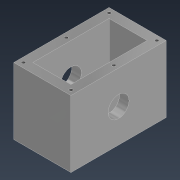
# Autodesk Inventor part: P016-Carter_corps
Saved by Autodesk Inventor 2021.3 (Build 253353000, 353)
## iProperties
Created: 2022-04-01
Part Number: P016-Carter_corps
Material: Aluminium
Document SubType Name: Modeling
Designer: remi
Density: 2.7 g/cm^3
Appearance: Aluminum - Dark
Author: remi
Autodesk Inventor part; units mm, degrees
ref_plane "YZ Plane" through (0, 0, 0) normal (1, 0, 0) x (0, 1, 0)
ref_plane "XZ Plane" through (0, 0, 0) normal (0, 1, 0) x (-1, 0, 0)
ref_plane "XY Plane" through (0, 0, 0) normal (0, 0, 1) x (1, 0, 0)
sketch "Sketch2" plane through (0, 0, 0) normal (0, 0, 1) x (1, 0, 0)
  line L0 (-30, -50) -> (30, -50)
  line L1 (30, -50) -> (30, 50)
  line L2 (30, 50) -> (-30, 50)
  line L3 (-30, 50) -> (-30, -50)
  line L4 (-30, -50) -> (30, 50) construction
  line L5 (30, -50) -> (-30, 50) construction
  line L6 (20, -40) -> (-20, -40)
  line L7 (-20, -40) -> (-20, 40)
  line L8 (-20, 40) -> (20, 40)
  line L9 (20, 40) -> (20, -40)
  line L10 (20, -40) -> (-20, 40) construction
  line L11 (-20, -40) -> (20, 40) construction
  point P0 (0, 0)
  dimension "d0" = 60
  dimension "d1" = 10
  dimension "d2" = 10
  dimension "d3" = 80
  constraints: 24 end point, 4 midpoint, 4 parallel, 2 horizontal, 2 perpendicular
  measures "d0" distance of L1.end L2.end
  measures "d1" distance between parallel lines of L3 L7
  measures "d2" distance between parallel lines of L2 L8
  measures "d3" distance of L6.end L7.end
extrude "Extrusion1" add sketch "Sketch2" along normal blind 60
sketch "Sketch3" plane through (0, 0, 0) normal (0, 0, -1) x (-1, 0, 0)
  line L0 (-30, -50) -> (-30, 50) projected
  line L1 (30, -50) -> (-30, -50) projected
  line L2 (30, 50) -> (30, -50) projected
  line L3 (-30, 50) -> (30, 50) projected
  line L4 (-20, -40) -> (20, -40) construction
  line L5 (-20, 40) -> (-20, -40) construction
  line L6 (20, 40) -> (-20, 40) construction
  line L7 (20, -40) -> (20, 40) construction
  point P0 (0, 0)
extrude "Extrusion2" add sketch "Sketch3" along normal blind 10
sketch "Sketch4" plane through (30, -50, 60) normal (1, 0, 0) x (0, 0, -1)
  line L0 (70, 100) -> (0, 100) construction
  line L1 (0, 0) -> (0, 100) construction
  line L2 (0, 0) -> (70, 0) construction
  line L3 (70, 100) -> (70, 0) construction
  line L4 (70, 0) -> (0, 100) construction
  line L5 (0, 0) -> (70, 100) construction
  point P0 (60, 50)
  point P1 (35, 50)
  constraints: 4 end point, 2 midpoint
hole "Hole1" at (30, 0, 25) direction (-1, 0, 0) diameter 22 end through all
sketch "Sketch5" plane through (0, 0, 60) normal (0, 0, 1) x (1, 0, 0)
  line L0 (30, -50) -> (30, 50) construction
  line L1 (30, 50) -> (-30, 50) construction
  line L2 (-30, 50) -> (-30, -50) construction
  line L3 (-30, -50) -> (30, -50) construction
  line L4 (20, -40) -> (-20, -40) construction
  line L5 (-20, -40) -> (-20, 40) construction
  line L6 (-20, 40) -> (20, 40) construction
  line L7 (20, 40) -> (20, -40) construction
  line L8 (-25, -45) -> (25, -45) construction
  line L9 (25, -45) -> (25, 45) construction
  line L10 (25, 45) -> (-25, 45) construction
  line L11 (-25, 45) -> (-25, -45) construction
  line L12 (-25, -45) -> (25, 45) construction
  line L13 (25, -45) -> (-25, 45) construction
  line L14 (-20, 40) -> (-25, 45) construction
  line L15 (-25, 45) -> (-30, 50) construction
  line L16 (-42, 0) -> (42, 0) construction
  point P0 (0, 0)
  point P1 (-25, 0)
  point P2 (25, 0)
  constraints: 16 end point, 4 coincident, 4 midpoint, 2 collinear, 2 parallel, 2 point on line, 1 horizontal, 1 perpendicular
hole "Hole2" at (25, -45, 60) at (-25, -45, 60) at (-25, 45, 60) at (25, 45, 60) at (-25, 0, 60) at (25, 0, 60) direction (0, 0, -1) diameter 3.242 depth 10 thread size "M4x0.7" class "6H" standard "ISO Metric profile"
equation "\"d2\" = d1"
body "Solid1"
